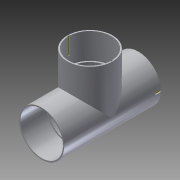
# Autodesk Inventor part: 0pvc_T_2in
Saved by Autodesk Inventor 2014 (Build 180170000, 170)
## iProperties
Company: HERA Project
Created: 2013-06-12
Part Number: 0pvc_T_2in
Material: PVC-Piping
Document SubType Name: Modeling
Designer: David DeBoer
Density: 1.4 g/cm^3
Description: Support PVC T
Mass: 203.947 g
Surface Area: 804.661 cm^2
Volume: 145.677 cm^3
Appearance: Smooth - White
Author: David DeBoer
Title: sup
Autodesk Inventor part; units mm, degrees
ref_plane "XZ Plane" through (0, 0, 0) normal (0, 1, 0) x (-1, 0, 0)
sketch "Sketch1" plane through (0, 0, 0) normal (0, 0, 1) x (1, 0, 0)
  circle A0 centre (0, 0) radius 33.45
  dimension "d0" = 66.9
  constraints: 1 centre point, 1 coincident
  measures "d0" diameter of A0
extrude "mainBody" add sketch "Sketch1" along normal blind 143.5
sketch "Sketch10" plane through (0, 0, 143.5) normal (0, 0, 1) x (1, 0, 0)
  circle A0 centre (0, 0) radius 30.1625 projected
  circle A1 centre (0, 0) radius 33.45 projected
  point P0 (0, 33.45)
  constraints: 1 vertical alignment, 1 other
ref_plane "Work Plane5" through (0, 33.45, 143.5) normal (0, 1, 0) x (-1, 0, 0)
sketch "Sketch11" plane through (0, 33.45, 143.5) normal (0, 1, 0) x (-1, 0, 0)
  circle A0 centre (0, -71.75) radius 33.45
  line L0 (33.45, 0) -> (-33.45, 0) projected
  point P0 (0, -143.5)
  dimension "d29" = 71.75
  dimension "d30" = 66.9
  constraints: 1 centre point
  measures "d29" distance from line of A0.centre L0
  measures "d30" diameter of A0
extrude "TBody" add sketch "Sketch11" along normal blind 40 and the other way blind 31.75
sketch "Sketch12" plane through (0, 73.45, 71.75) normal (0, 1, 0) x (1, 0, 0)
  circle A0 centre (0, 0) radius 33.45 projected
  circle A1 centre (0, 0) radius 31.6
  point P0 (0, 71.75)
  dimension "d35" = 63.2
  constraints: 1 centre point, 1 coincident
  measures "d35" diameter of A1
extrude "TSocket" cut sketch "Sketch12" against normal blind 38.3 contours A1
sketch "Sketch13" plane through (0, 35.15, 71.75) normal (0, 1, 0) x (1, 0, 0)
  circle A0 centre (0, 0) radius 31.6 projected
  circle A1 centre (0, 0) radius 29.5
  point P0 (0, 71.75)
  dimension "d39" = 59
  constraints: 1 centre point, 1 coincident
  measures "d39" diameter of A1
extrude "TTube" cut sketch "Sketch13" against normal blind 38.1 contours A1
sketch "Sketch14" plane through (0, 0, 143.5) normal (0, 0, 1) x (1, 0, 0)
  circle A0 centre (0, 0) radius 33.45 projected
  circle A1 centre (0, 0) radius 29.5
  dimension "d43" = 59
  constraints: 1 centre point, 1 coincident
  measures "d43" diameter of A1
extrude "mainTube" cut sketch "Sketch14" against normal blind 177.8 contours A1
sketch "Sketch15" plane through (0, 0, 143.5) normal (0, 0, 1) x (1, 0, 0)
  circle A0 centre (0, 0) radius 29.5 projected
  circle A1 centre (0, 0) radius 33.45 projected
  circle A2 centre (0, 0) radius 31.6
  dimension "d47" = 63.2
  constraints: 1 centre point, 1 coincident
  measures "d47" diameter of A2
extrude "mainSocket1" cut sketch "Sketch15" against normal blind 38.3 contours A2
sketch "Sketch16" plane through (0, 0, 0) normal (0, 0, -1) x (-1, 0, 0)
  circle A0 centre (0, 0) radius 29.5 projected
  circle A1 centre (0, 0) radius 33.45 projected
  circle A2 centre (0, 0) radius 31.6
  dimension "d51" = 63.2
  constraints: 1 centre point, 1 coincident
  measures "d51" diameter of A2
extrude "mainSocket2" cut sketch "Sketch16" against normal blind 38.3 contours A2
sketch "Sketch24" plane through (0, 73.45, 71.75) normal (0, 1, 0) x (1, 0, 0)
  circle A0 centre (0, 0) radius 31.6 projected
  line L0 (-31.6, 0) -> (31.6, 0) construction
  line L1 (0, 31.6) -> (0, -31.6) construction
  line L2 (-32.3825, -1.27) -> (-28.3825, -1.27)
  line L3 (-28.3825, -1.27) -> (-28.3825, 1.27)
  line L4 (-28.3825, 1.27) -> (-32.3825, 1.27)
  line L5 (-32.3825, 1.27) -> (-32.3825, -1.27)
  line L6 (-32.3825, 0) -> (-28.3825, 0) construction
  line L7 (32.3825, -1.27) -> (28.3825, -1.27)
  line L8 (28.3825, -1.27) -> (28.3825, 1.27)
  line L9 (28.3825, 1.27) -> (32.3825, 1.27)
  line L10 (32.3825, 1.27) -> (32.3825, -1.27)
  line L11 (32.3825, 0) -> (28.3825, 0) construction
  point P0 (0, 71.75)
  dimension "d72" = 4
  dimension "d75" = 2.54
  constraints: 24 end point, 6 symmetric about line, 4 point on circle, 2 horizontal, 2 midpoint, 2 parallel, 2 perpendicular, 1 collinear
  measures "d72" distance of L4.end L3.end
  measures "d75" distance of L2.end L3.end
extrude "Extrusion20" cut sketch "Sketch24" against normal blind 25.4 contours A0 L7 L8 L9 | A0 L9 L10 L7 | L4 L3 L2 A0 | A0 L2 L5 L4
ref_plane "Work Plane6" through (32, 0, 0) normal (1, 0, 0) x (0, 1, 0)
sketch "Sketch27" plane through (32, 0, 0) normal (1, 0, 0) x (0, 1, 0)
  line L0 (-1.5232, -1.2223) -> (1.5232, -1.2223)
  line L1 (1.5232, -1.2223) -> (1.5232, 8.0295)
  line L2 (1.5232, 8.0295) -> (-1.5232, 8.0295)
  line L3 (-1.5232, 8.0295) -> (-1.5232, -1.2223)
  point P0 (0, 0)
  constraints: 8 end point, 2 parallel, 1 horizontal, 1 perpendicular
extrude "Extrusion22" cut sketch "Sketch27" along normal blind 25.4
equation "\"d1\" = length"
equation "\"d29\" = 0.5 * length"
equation "\"length\" = 143.5"
body "Solid1"
